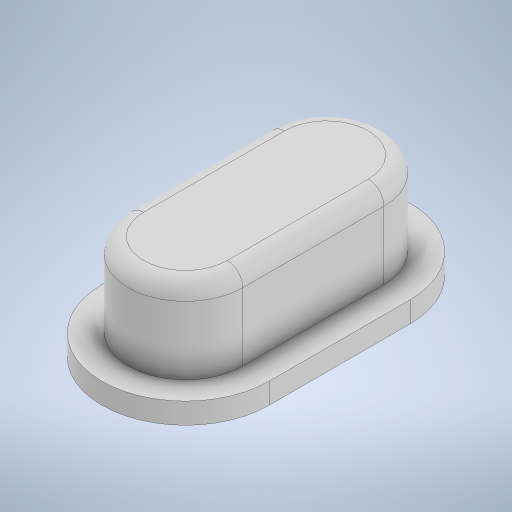
# Autodesk Inventor part: Button
Saved by Autodesk Inventor 2023 (Build 270158000, 158)
## iProperties
Created: 2023-03-17
Part Number: Button
Material: Generic
Document SubType Name: Modeling
Designer: nigel
Density: 1 g/cm^3
Appearance: Default
Author: nigel
Autodesk Inventor part; units mm, degrees
ref_plane "YZ Plane" through (0, 0, 0) normal (1, 0, 0) x (0, 1, 0)
ref_plane "XZ Plane" through (0, 0, 0) normal (0, 1, 0) x (-1, 0, 0)
ref_plane "XY Plane" through (0, 0, 0) normal (0, 0, 1) x (1, 0, 0)
sketch "Sketch1" plane through (0, 0, 0) normal (0, 1, 0) x (-1, 0, 0)
  line L0 (0, 1.35) -> (0, -1.35) construction
  line L1 (-1.1, 1.35) -> (-1.1, -1.35)
  line L2 (1.1, -1.35) -> (1.1, 1.35)
  arc A0 (1.1, 1.35) -> (-1.1, 1.35) centre (0, 1.35) ccw
  arc A1 (-1.1, -1.35) -> (1.1, -1.35) centre (0, -1.35) ccw
  line L3 (1.6, 1.35) -> (1.6, -1.35)
  arc A2 (-1.6, -1.35) -> (1.6, -1.35) centre (0, -1.35) ccw
  line L4 (-1.6, -1.35) -> (-1.6, 1.35)
  arc A3 (1.6, 1.35) -> (-1.6, 1.35) centre (0, 1.35) ccw
  point P0 (0, 0)
  dimension "d0" = 2.7
  dimension "d1" = 2.2
  dimension "d2" = 0.5
  constraints: 12 end point, 8 point on circle, 4 centre point, 4 tangent, 2 parallel, 1 midpoint, 1 vertical, 3 other
  measures "d0" distance of L0.start L0.end
  measures "d1" distance between parallel lines of L1 L2
  measures "d2" distance between parallel lines of L2 L3
extrude "Extrusion1" add sketch "Sketch1" along normal blind 2 contours A0 L2 A1 L1
extrude "Extrusion2" add sketch "Sketch1" along normal blind 0.4
fillet "Fillet1" radius 0.3 4 edges at (0, 2, -2.45) (-1.1, 2, 0) (0, 2, 2.45) (1.1, 2, 0)
body "Solid1"
